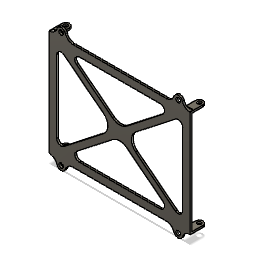
Powersupplybracket (Autodesk Fusion 360 design; units mm, degrees)
Autodesk Fusion 360 part; units mm, degrees
sketch "Skizze1" plane through (0, 0, 0) normal (0, 1, 0) x (1, 0, 0)
  line L0 (150, -12.5) -> (0, -12.5)
  circle A0 centre (150, 0) radius 2.25
  line L1 (-4.25, -12.5) -> (-4.25, 0)
  arc A1 (4.25, 0) -> (-4.25, 0) centre (0, 0) ccw
  line L2 (4.25, 0) -> (4.25, -12.5)
  circle A2 centre (0, 0) radius 2.25
  line L3 (0, -12.5) -> (-4.25, -12.5)
  line L4 (145.75, 0) -> (145.75, -12.5)
  line L5 (154.25, -12.5) -> (154.25, 0)
  arc A3 (154.25, 0) -> (145.75, 0) centre (150, 0) ccw
  line L6 (150, -12.5) -> (154.25, -12.5)
  line L7 (-4.25, -12.5) -> (154.25, -12.5)
  line L8 (154.25, -12.5) -> (154.25, -14.5)
  line L9 (154.25, -14.5) -> (-4.25, -14.5)
  line L10 (-4.25, -14.5) -> (-4.25, -12.5)
  dimension "d1" = 150
  dimension "d2" = 12.5
  dimension "d4" = 4.5
  dimension "d7" = 2
  constraint horizontal L0
  constraint tangent L1 A1
  constraint tangent A1 L2
  constraint perpendicular L1 L3
  constraint coincident L0 L2.end
  constraint horizontal L7
  constraint vertical L8
  constraint horizontal L9
  constraint vertical L10
  measures "d1" distance of A1.centre A0.centre
  measures "d2" distance of A1.centre L0.end
  measures "d4" diameter of A0
  measures "d7" distance of L1.start L9.end
extrude "Extrusion1" add sketch "Skizze1" along normal blind 2 makes body 1
extrude "Extrusion2" add sketch "Skizze1" against normal blind 115.4 contours L0 L3 L6 L7 L8 L9 L10 bodies 1
sketch "Skizze2" plane through (0, -115.4, 0) normal (0, -1, 0) x (1, 0, 0)
  line L0 (154.25, 14.5) -> (-4.25, 14.5)
  line L1 (-4.25, 14.5) -> (-4.25, 12.5)
  line L2 (-4.25, 12.5) -> (154.25, 12.5)
  line L3 (154.25, 12.5) -> (154.25, 14.5)
  circle A0 centre (150, 0) radius 2.25
  circle A1 centre (0, 0) radius 2.25
  line L4 (-4.25, 14.5) -> (154.25, 14.5)
  line L5 (-4.25, 0) -> (-4.25, 14.5)
  arc A2 (-4.25, 0) -> (4.25, 0) centre (0, 0) ccw
  line L6 (4.25, 12.5) -> (4.25, 0)
  line L7 (145.75, 12.5) -> (4.25, 12.5)
  line L8 (145.75, 0) -> (145.75, 12.5)
  arc A3 (145.75, 0) -> (154.25, 0) centre (150, 0) ccw
  line L9 (154.25, 14.5) -> (154.25, 0)
extrude "Extrusion3" add sketch "Skizze2" along normal blind 2 bodies 1
sketch "Skizze3" plane through (0, 0, 12.5) normal (0, 0, -1) x (-1, 0, 0)
  line L0 (-4.25, 0) -> (-4.25, 2)
  line L1 (-145.75, 2) -> (-145.75, 0)
  line L2 (-145.75, 0) -> (-154.25, 0)
  line L3 (-154.25, 0) -> (-154.25, -115.4)
  line L4 (-154.25, -115.4) -> (-145.75, -115.4)
  line L5 (-145.75, -115.4) -> (-145.75, -117.4)
  line L6 (-145.75, -117.4) -> (-4.25, -117.4)
  line L7 (-4.25, -117.4) -> (-4.25, -115.4)
  line L8 (-4.25, -115.4) -> (4.25, -115.4)
  line L9 (4.25, -115.4) -> (4.25, 0)
  line L10 (4.25, 0) -> (-4.25, 0)
  line L11 (-154.25, -117.4) -> (4.25, -117.4)
  line L12 (-154.25, -117.4) -> (-154.25, 2)
  line L13 (4.25, 2) -> (-154.25, 2)
  line L14 (4.25, -117.4) -> (4.25, 2)
  line L15 (-154.25, 0) -> (-4.25, -117.4)
  line L16 (-145.75, -117.4) -> (4.25, 0)
  line L17 (-154.25, 0) -> (-145.75, 0)
  line L18 (-145.75, 2) -> (-145.75, 0)
  line L19 (-4.25, 2) -> (-4.25, 0)
  line L20 (4.25, 0) -> (-4.25, 0)
  line L21 (-145.75, -117.4) -> (-145.75, 2)
  line L22 (-154.25, -115.4) -> (-4.25, 2)
  line L23 (4.25, -115.4) -> (-145.75, 2)
  line L24 (-4.25, -117.4) -> (-4.25, 2)
  line L25 (4.25, 2) -> (-154.25, 2)
  line L26 (-154.25, 2) -> (-154.25, -6.5)
  line L27 (-154.25, -6.5) -> (4.25, -6.5)
  line L28 (4.25, -6.5) -> (4.25, 2)
  line L29 (4.25, -117.4) -> (-154.25, -117.4)
  line L30 (-154.25, -117.4) -> (-154.25, -108.9)
  line L31 (-154.25, -108.9) -> (4.25, -108.9)
  line L32 (4.25, -108.9) -> (4.25, -117.4)
  point P0 (4.25, -117.4)
  point P1 (-154.25, -117.4)
  dimension "d20" = 8.5
  dimension "d21" = 8.5
  constraint coincident L2.end L3.start
  constraint coincident L6.end L7.start
  constraint coincident L1.start L18.start
  constraint coincident L0.end L19.start
  constraint coincident L5.end L6.start
  constraint coincident L9.end L10.start
  constraint coincident L1.end L2.start
  constraint coincident L0.start L10.end
  constraint coincident L3.end L4.start
  constraint coincident L8.end L9.start
  constraint horizontal L25
  constraint vertical L26
  constraint horizontal L27
  constraint vertical L28
  constraint coincident L3 L26.end
  constraint coincident L13.start L14.end
  constraint horizontal L29
  constraint vertical L30
  constraint horizontal L31
  constraint vertical L32
  constraint coincident L3 L30.end
  constraint coincident P0 L11.end
  measures "d20" distance of L13.start L27.end
  measures "d21" distance of P0 L31.end
extrude "Extrusion5" cut sketch "Skizze3" against normal blind 55 contours L22 L23 L27 | L16 L23 L24 | L15 L21 L22 | L15 L16 L31 bodies 1
fillet "Abrundung3" radius 12.5 4 edges at (75, -53.3737, 13.5) (69.4723, -57.7, 13.5) (80.5277, -57.7, 13.5) (75, -62.0263, 13.5) on bodies 1
fillet "Abrundung4" radius 5 8 edges at (134.8897, -6.5, 13.5) (145.75, -6.6527, 13.5) (15.1103, -108.9, 13.5) (4.25, -108.7473, 13.5) (4.25, -6.6527, 13.5) (15.1103, -6.5, 13.5) (145.75, -108.7473, 13.5) (134.8897, -108.9, 13.5) on bodies 1
sketch "Skizze4" plane through (0, 0, 14.5) normal (0, 0, 1) x (1, 0, 0)
  line L0 (29.6112, -6.5) -> (120.3888, -6.5)
  arc A0 (123.4705, -15.4374) -> (120.3888, -6.5) centre (120.3888, -11.5) ccw
  line L1 (123.4705, -15.4374) -> (82.7042, -47.3438)
  arc A1 (67.2958, -47.3438) -> (82.7042, -47.3438) centre (75, -37.5003) ccw
  line L2 (67.2958, -47.3438) -> (26.5295, -15.4374)
  arc A2 (29.6112, -6.5) -> (26.5295, -15.4374) centre (29.6112, -11.5) ccw
  line L3 (26.5295, -99.9626) -> (67.2958, -68.0562)
  arc A3 (82.7042, -68.0562) -> (67.2958, -68.0562) centre (75, -77.8997) ccw
  line L4 (82.7042, -68.0562) -> (123.4705, -99.9626)
  arc A4 (120.3888, -108.9) -> (123.4705, -99.9626) centre (120.3888, -103.9) ccw
  line L5 (120.3888, -108.9) -> (29.6112, -108.9)
  arc A5 (26.5295, -99.9626) -> (29.6112, -108.9) centre (29.6112, -103.9) ccw
  line L6 (12.3317, -12.9779) -> (56.8954, -47.8565)
  arc A6 (56.8954, -67.5435) -> (56.8954, -47.8565) centre (49.1912, -57.7) ccw
  line L7 (56.8954, -67.5435) -> (12.3317, -102.4221)
  arc A7 (4.25, -98.4847) -> (12.3317, -102.4221) centre (9.25, -98.4847) ccw
  line L8 (4.25, -98.4847) -> (4.25, -16.9153)
  arc A8 (12.3317, -12.9779) -> (4.25, -16.9153) centre (9.25, -16.9153) ccw
  line L9 (93.1046, -47.8565) -> (137.6683, -12.9779)
  arc A9 (145.75, -16.9153) -> (137.6683, -12.9779) centre (140.75, -16.9153) ccw
  line L10 (145.75, -16.9153) -> (145.75, -98.4847)
  arc A10 (137.6683, -102.4221) -> (145.75, -98.4847) centre (140.75, -98.4847) ccw
  line L11 (137.6683, -102.4221) -> (93.1046, -67.5435)
  arc A11 (93.1046, -47.8565) -> (93.1046, -67.5435) centre (100.8088, -57.7) ccw
  line L12 (154.25, -117.4) -> (154.25, 2)
  line L13 (154.25, 2) -> (-4.25, 2)
  line L14 (-4.25, 2) -> (-4.25, -117.4)
  line L15 (-4.25, -117.4) -> (154.25, -117.4)
  arc A12 (120.3888, -108.9) -> (123.4705, -99.9626) centre (120.3888, -103.9) ccw
  line L16 (29.6112, -108.9) -> (120.3888, -108.9)
  arc A13 (137.6683, -102.4221) -> (145.75, -98.4847) centre (140.75, -98.4847) ccw
  line L17 (93.1046, -67.5435) -> (137.6683, -102.4221)
  arc A14 (29.6112, -6.5) -> (26.5295, -15.4374) centre (29.6112, -11.5) ccw
  line L18 (120.3888, -6.5) -> (29.6112, -6.5)
  arc A15 (12.3317, -12.9779) -> (4.25, -16.9153) centre (9.25, -16.9153) ccw
  line L19 (56.8954, -47.8565) -> (12.3317, -12.9779)
  arc A16 (4.25, -98.4847) -> (12.3317, -102.4221) centre (9.25, -98.4847) ccw
  line L20 (4.25, -16.9153) -> (4.25, -98.4847)
  arc A17 (26.5295, -99.9626) -> (29.6112, -108.9) centre (29.6112, -103.9) ccw
  line L21 (67.2958, -68.0562) -> (26.5295, -99.9626)
  arc A18 (145.75, -16.9153) -> (137.6683, -12.9779) centre (140.75, -16.9153) ccw
  line L22 (145.75, -98.4847) -> (145.75, -16.9153)
  arc A19 (123.4705, -15.4374) -> (120.3888, -6.5) centre (120.3888, -11.5) ccw
  line L23 (82.7042, -47.3438) -> (123.4705, -15.4374)
  arc A20 (82.7042, -68.0562) -> (67.2958, -68.0562) centre (75, -77.8997) ccw
  line L24 (123.4705, -99.9626) -> (82.7042, -68.0562)
  arc A21 (93.1046, -47.8565) -> (93.1046, -67.5435) centre (100.8088, -57.7) ccw
  line L25 (137.6683, -12.9779) -> (93.1046, -47.8565)
  arc A22 (56.8954, -67.5435) -> (56.8954, -47.8565) centre (49.1912, -57.7) ccw
  line L26 (12.3317, -102.4221) -> (56.8954, -67.5435)
  arc A23 (67.2958, -47.3438) -> (82.7042, -47.3438) centre (75, -37.5003) ccw
  line L27 (26.5295, -15.4374) -> (67.2958, -47.3438)
  line L28 (154.25, -115.4) -> (154.25, -117.4)
  line L29 (145.75, -117.4) -> (154.25, -117.4)
  line L30 (-4.25, -117.4) -> (4.25, -117.4)
  line L31 (-4.25, -115.4) -> (-4.25, -117.4)
  line L32 (4.25, -117.4) -> (145.75, -117.4)
  line L33 (-4.25, 0) -> (-4.25, 2)
  line L34 (-4.25, 0) -> (-4.25, -115.4)
  line L35 (4.25, 2) -> (-4.25, 2)
  line L36 (145.75, 2) -> (4.25, 2)
  line L37 (154.25, 0) -> (154.25, -115.4)
  line L38 (154.25, 2) -> (145.75, 2)
  line L39 (154.25, 0) -> (154.25, 2)
  line L40 (145.75, -117.4) -> (135.75, -117.4)
  line L41 (135.75, -117.4) -> (135.75, -127.4)
  line L42 (135.75, -127.4) -> (145.75, -127.4)
  line L43 (145.75, -127.4) -> (145.75, -117.4)
  line L44 (4.25, -117.4) -> (14.25, -117.4)
  line L45 (14.25, -117.4) -> (14.25, -127.4)
  line L46 (14.25, -127.4) -> (4.25, -127.4)
  line L47 (4.25, -127.4) -> (4.25, -117.4)
  line L48 (4.25, 2) -> (14.25, 2)
  line L49 (14.25, 2) -> (14.25, 12)
  line L50 (14.25, 12) -> (4.25, 12)
  line L51 (4.25, 12) -> (4.25, 2)
  line L52 (145.75, 2) -> (135.75, 2)
  line L53 (135.75, 2) -> (135.75, 12)
  line L54 (135.75, 12) -> (145.75, 12)
  line L55 (145.75, 12) -> (145.75, 2)
  circle A24 centre (140.75, -122.4) radius 2.5
  circle A25 centre (9.25, -122.4) radius 2.5
  circle A26 centre (140.75, 7) radius 2.5
  circle A27 centre (9.25, 7) radius 2.5
  dimension "d28" = 10
  dimension "d29" = 10
  dimension "d30" = 10
  dimension "d31" = 10
  dimension "d32" = 10
  dimension "d33" = 10
  dimension "d34" = 10
  dimension "d35" = 10
  dimension "d36" = 5
  dimension "d37" = 5
  dimension "d38" = 5
  dimension "d39" = 5
  constraint horizontal L40
  constraint vertical L41
  constraint horizontal L42
  constraint vertical L43
  constraint coincident L29.start L32.end
  constraint horizontal L44
  constraint vertical L45
  constraint horizontal L46
  constraint vertical L47
  constraint coincident L30.end L32.start
  constraint horizontal L48
  constraint vertical L49
  constraint horizontal L50
  constraint vertical L51
  constraint coincident L35.start L36.end
  constraint horizontal L52
  constraint vertical L53
  constraint horizontal L54
  constraint vertical L55
  constraint coincident L36.start L38.end
  measures "d28" distance of L29.start L40.end
  measures "d29" distance of L29.start L42.end
  measures "d30" distance of L30.end L44.end
  measures "d31" distance of L30.end L46.end
  measures "d32" distance of L35.start L48.end
  measures "d33" distance of L35.start L50.end
  measures "d34" distance of L36.start L52.end
  measures "d35" distance of L36.start L54.end
  measures "d36" diameter of A24
  measures "d37" diameter of A25
  measures "d38" diameter of A26
  measures "d39" diameter of A27
extrude "Extrusion6" add sketch "Skizze4" against normal blind 2 contours L15 L32 L40 L41 L42 L43 | L15 L32 L44 L45 L46 L47 | L13 L36 L52 L53 L54 L55 | L13 L36 L48 L49 L50 L51 bodies 1
fillet "Abrundung5" radius 5 8 edges at (14.25, 12, 13.5) (4.25, 12, 13.5) (145.75, 12, 13.5) (135.75, 12, 13.5) (145.75, -127.4, 13.5) (135.75, -127.4, 13.5) (4.25, -127.4, 13.5) (14.25, -127.4, 13.5) on bodies 1
fillet "Abrundung6" radius 8.5 8 edges at (4.25, 2, 13.5) (14.25, 2, 13.5) (135.75, 2, 13.5) (145.75, 2, 13.5) (145.75, -117.4, 13.5) (135.75, -117.4, 13.5) (4.25, -117.4, 13.5) (14.25, -117.4, 13.5) on bodies 1
fillet "Abrundung7" radius 2 4 edges at (149.7692, 2, 12.5) (0.2308, 2, 12.5) (0.2308, -117.4, 12.5) (149.7692, -117.4, 12.5) on bodies 1
copy_body "Körper->Berechn1" bodies 1 removing the originals makes body 2 in component "Component"
component "Component" placed x (1, 0, 0) y (0, 1, 0) z (0, 0, 1) at (0, 0, 0)
